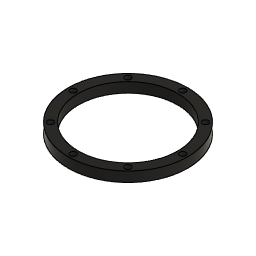
筒固定具 (Autodesk Fusion 360 design; units mm, degrees)
Autodesk Fusion 360 part; units mm, degrees
note: some values were not read from the file. Set by a fixed rule: which sketch regions a step uses.
sketch "スケッチ1" plane through (0, 0, 0) normal (0, 0, 1) x (1, 0, 0)
  circle A0 centre (0, 0) radius 25
  circle A1 centre (0, 0) radius 27.5
  dimension "d1" = 55
  constraint coincident A0.centre A1.centre
  measures "d1" diameter of A1
extrude "押し出し1" add sketch "スケッチ1" along normal blind 5
sketch "スケッチ2" plane through (0, 0, 5) normal (0, 0, 1) x (-1, 0, 0)
  circle A0 centre (0, 0) radius 25
  circle A1 centre (0, 0) radius 27.5
  circle A2 centre (0, 0) radius 30
  constraint coincident A0.centre A1.centre
extrude "押し出し2" add sketch "スケッチ2" against normal blind 5 contours A2
sketch "スケッチ3" plane through (0, 0, 5) normal (0, 0, 1) x (-1, 0, 0)
  circle A0 centre (0, 0) radius 30
  circle A1 centre (0, 0) radius 25
  circle A2 centre (0, 0) radius 27.5
  circle A3 centre (-27.5, 0) radius 1.5
  circle A4 centre (-19.4454, -19.4454) radius 1.5
  circle A5 centre (0, -27.5) radius 1.5
  circle A6 centre (19.4454, -19.4454) radius 1.5
  circle A7 centre (27.5, 0) radius 1.5
  circle A8 centre (19.4454, 19.4454) radius 1.5
  circle A9 centre (0, 27.5) radius 1.5
  circle A10 centre (-19.4454, 19.4454) radius 1.5
  dimension "d6" = 55
  dimension "d7" = 3
  dimension "d9" = 360
  constraint coincident A0.centre A1.centre
  constraint coincident A2 A3.centre
  measures "d6" diameter of A2
  measures "d7" diameter of A3
extrude "押し出し3" cut sketch "スケッチ3" against normal blind 6 contours A2 A7 | A2 A7 | A2 A8 | A2 A8 | A2 A6 | A2 A6 | A2 A9 | A2 A9 | A2 A5 | A2 A5 | A2 A10 | A2 A10 | A2 A4 | A2 A4 | A2 A3 | A2 A3
